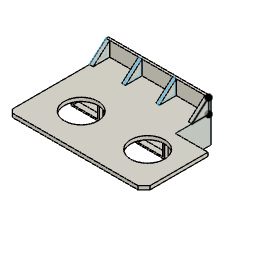
Magneto+Cooler+Gehäuse (Autodesk Fusion 360 design; units mm, degrees)
Autodesk Fusion 360 part; units mm, degrees
sketch "Skizze1" plane through (0, 0, 0) normal (0, 1, 0) x (1, 0, 0)
  line L0 (0, 0) -> (85, 0)
  line L1 (85, 0) -> (85, -25)
  line L2 (85, -25) -> (0, -25)
  line L3 (0, -25) -> (0, 0)
  line L4 (85, 0) -> (85, -10)
  line L5 (5, -10) -> (17, -10)
  line L6 (17, -10) -> (17, -19)
  line L7 (17, -19) -> (5, -19)
  line L8 (5, -19) -> (5, -10)
  line L9 (32, -19) -> (20, -19)
  line L10 (20, -19) -> (20, -10)
  line L11 (20, -10) -> (32, -10)
  line L12 (32, -10) -> (32, -19)
  line L13 (47, -19) -> (35, -19)
  line L14 (35, -19) -> (35, -10)
  line L15 (35, -10) -> (47, -10)
  line L16 (47, -10) -> (47, -19)
  line L17 (62, -19) -> (50, -19)
  line L18 (50, -19) -> (50, -10)
  line L19 (50, -10) -> (62, -10)
  line L20 (62, -10) -> (62, -19)
  line L21 (82, -19) -> (70, -19)
  line L22 (70, -19) -> (70, -10)
  line L23 (70, -10) -> (82, -10)
  line L24 (82, -10) -> (82, -19)
  line L25 (6.5, -11.5) -> (15.5, -11.5)
  line L26 (15.5, -11.5) -> (15.5, -17.5)
  line L27 (15.5, -17.5) -> (6.5, -17.5)
  line L28 (6.5, -17.5) -> (6.5, -11.5)
  line L29 (21.5, -11.5) -> (30.5, -11.5)
  line L30 (30.5, -11.5) -> (30.5, -17.5)
  line L31 (30.5, -17.5) -> (21.5, -17.5)
  line L32 (21.5, -17.5) -> (21.5, -11.5)
  line L33 (51.5, -11.5) -> (60.5, -11.5)
  line L34 (60.5, -11.5) -> (60.5, -17.5)
  line L35 (60.5, -17.5) -> (51.5, -17.5)
  line L36 (51.5, -17.5) -> (51.5, -11.5)
  line L37 (36.5, -11.5) -> (45.5, -11.5)
  line L38 (45.5, -11.5) -> (45.5, -17.5)
  line L39 (45.5, -17.5) -> (36.5, -17.5)
  line L40 (36.5, -17.5) -> (36.5, -11.5)
  line L41 (71.5, -11.5) -> (80.5, -11.5)
  line L42 (80.5, -11.5) -> (80.5, -17.5)
  line L43 (80.5, -17.5) -> (71.5, -17.5)
  line L44 (71.5, -17.5) -> (71.5, -11.5)
  dimension "d1" = 85
  dimension "d2" = 25
  dimension "d3" = 10
  dimension "d4" = 12
  dimension "d5" = 9
  dimension "d9" = 45
  dimension "d10" = 0
  dimension "d13" = 20
  dimension "d14" = 0
  dimension "d16" = 1.5
  dimension "d17" = 1.5
  dimension "d18" = 1.5
  dimension "d19" = 1.5
  dimension "d20" = 1.5
  constraint horizontal L0
  constraint vertical L1
  constraint horizontal L2
  constraint vertical L3
  constraint coincident L0.start L3.end
  constraint perpendicular L0 L4
  constraint horizontal L5
  constraint vertical L6
  constraint horizontal L7
  constraint vertical L8
  measures "d1" distance of L0.start L0.end
  measures "d2" distance of L0.start L2.end
  measures "d3" distance of L0.end L4.end
  measures "d4" distance of L5.start L5.end
  measures "d5" distance of L5.start L7.end
extrude "Extrusion1" add sketch "Skizze1" along normal blind 3 contours L0 L1 L2 L3 L4
extrude "Extrusion2" add sketch "Skizze1" along normal blind 5 contours L5 L6 L7 L8 | L9 L10 L11 L12 | L13 L14 L15 L16 | L17 L18 L19 L20 | L21 L22 L23 L24
sketch "Skizze2" plane through (0, 0, 0) normal (0, 1, 0) x (1, 0, 0)
  line L0 (0, -25) -> (85, -25)
  line L1 (85, -25) -> (85, 0)
  line L2 (85, 0) -> (0, 0)
  line L3 (0, 0) -> (0, -25)
  line L4 (83.5, -1.5) -> (1.5, -1.5)
  line L5 (1.5, -1.5) -> (1.5, -23.5)
  line L6 (1.5, -23.5) -> (83.5, -23.5)
  line L7 (83.5, -23.5) -> (83.5, -1.5)
  point P0 (0, -25)
  point P1 (85, 0)
  dimension "d25" = -1.5
  constraint horizontal L0
  constraint vertical L1
  constraint horizontal L2
  constraint vertical L3
  constraint coincident P1 L1.end
  constraint coincident P0 L0.start
extrude "Extrusion3" add sketch "Skizze2" against normal blind 25
sketch "Skizze3" plane through (0, -25, 0) normal (0, -1, 0) x (1, 0, 0)
  line L0 (83.5, 23.5) -> (83.5, 1.5)
  line L1 (83.5, 1.5) -> (1.5, 1.5)
  line L2 (1.5, 1.5) -> (1.5, 23.5)
  line L3 (1.5, 23.5) -> (83.5, 23.5)
  line L4 (0, 25) -> (0, 0)
  line L5 (0, 0) -> (85, 0)
  line L6 (85, 0) -> (85, 25)
  line L7 (85, 25) -> (0, 25)
  line L8 (0, 25) -> (85, 25)
  line L9 (85, 25) -> (85, 0)
  line L10 (85, 0) -> (0, 0)
  line L11 (0, 0) -> (0, 25)
  constraint horizontal L8
  constraint vertical L9
  constraint horizontal L10
  constraint vertical L11
  constraint coincident L5.end L6.start
  constraint coincident L4.start L7.end
extrude "Extrusion4" add sketch "Skizze3" along normal blind 1.5 contours L0 L1 L2 L3 | L4 L5 L6 L7 L8 L9 L10 L11
sketch "Skizze4" plane through (0, -26.5, 0) normal (0, -1, 0) x (1, 0, 0)
  line L0 (0, 0) -> (85, 0)
  line L1 (85, 0) -> (85, 25)
  line L2 (85, 25) -> (0, 25)
  line L3 (0, 25) -> (0, 0)
  line L4 (3, 20) -> (22.8, 20)
  line L5 (22.8, 20) -> (22.8, 4.6)
  line L6 (22.8, 4.6) -> (3, 4.6)
  line L7 (3, 4.6) -> (3, 20)
  line L8 (4.45, 5.8) -> (21.35, 5.8)
  line L9 (21.35, 5.8) -> (21.35, 18.8)
  line L10 (21.35, 18.8) -> (4.45, 18.8)
  line L11 (4.45, 18.8) -> (4.45, 5.8)
  line L12 (76.8, 4.6) -> (57, 4.6)
  line L13 (76.8, 20) -> (76.8, 4.6)
  line L14 (58.45, 18.8) -> (58.45, 5.8)
  line L15 (57, 20) -> (76.8, 20)
  line L16 (75.35, 5.8) -> (75.35, 18.8)
  line L17 (75.35, 18.8) -> (58.45, 18.8)
  line L18 (57, 4.6) -> (57, 20)
  line L19 (58.45, 5.8) -> (75.35, 5.8)
  line L20 (109, 20) -> (109, 23)
  line L21 (109, 23) -> (0, 23)
  line L22 (109, 20) -> (0, 20)
  line L23 (0, 23) -> (0, 20)
  dimension "d30" = 19.8
  dimension "d31" = 15.4
  dimension "d33" = 16.9
  dimension "d34" = 13
  dimension "d36" = 19.8
  dimension "d37" = 15.4
  dimension "d38" = 16.9
  dimension "d39" = 13
  dimension "d40" = 52
  dimension "d41" = 3
  constraint horizontal L4
  constraint vertical L5
  constraint horizontal L6
  constraint vertical L7
  constraint horizontal L8
  constraint vertical L9
  constraint horizontal L10
  constraint vertical L11
  constraint horizontal L15
  constraint vertical L13
  constraint horizontal L12
  constraint vertical L18
  constraint horizontal L19
  constraint vertical L16
  constraint horizontal L17
  constraint vertical L14
  constraint coincident L3 L21.end
  constraint perpendicular L3 L21
  constraint coincident L3 L22.end
  constraint perpendicular L3 L22
  measures "d30" distance of L4.start L4.end
  measures "d31" distance of L4.start L6.end
  measures "d33" distance of L8.start L8.end
  measures "d34" distance of L8.start L10.end
  measures "d36" distance of L15.start L13.start
  measures "d37" distance of L15.start L12.end
  measures "d38" distance of L16.start L14.end
  measures "d39" distance of L14.end L14.start
  measures "d40" distance of L15.start L20.start
  measures "d41" distance of L20.start L20.end
extrude "Extrusion5" cut sketch "Skizze4" against normal blind 3 contours L8 L9 L10 L11 | L14 L16 L17 L19
extrude "Extrusion6" add sketch "Skizze4" along normal blind 3 contours L4 L5 L6 L7 L22 | L12 L13 L15 L18 L22
extrude "Extrusion7" add sketch "Skizze4" along normal blind 53 contours L1 L3 L4 L15 L21 L22 L23 | L1 L20 L21 L22
sketch "Skizze5" plane through (0, 0, 23) normal (0, 0, 1) x (-1, 0, 0)
  line L0 (-109, 26.5) -> (-85, 26.5)
  line L1 (-85, 26.5) -> (0, 26.5)
  line L2 (0, 26.5) -> (0, 79.5)
  line L3 (0, 79.5) -> (-109, 79.5)
  line L4 (-109, 79.5) -> (-109, 26.5)
  line L5 (-85, 26.5) -> (-85, 79.5)
  line L6 (-85, 26.5, 2) -> (-85, 79.5, 0)
  line L7 (-85, 26.5, 2) -> (-85, 26.5, 0)
  line L8 (0, 26.5) -> (0, 79.5)
  line L9 (0, 26.5, 2) -> (0, 79.5, 0)
  line L10 (0, 26.5, 2) -> (0, 26.5, 0)
  point P0 (-85, 26.5)
  point P1 (0, 26.5)
  point P2 (0, 26.5)
  constraint coincident P0 L0.end
  constraint coincident L3 L5.end
  constraint perpendicular L3 L5
  constraint coincident P2 P1
  constraint coincident L2.end L3.start
extrude "Extrusion8" add sketch "Skizze5" against normal blind 3 contours L2 L8 L9 L10 in plane through (0, 0, 23) normal (-1, 0, 0)
extrude "Extrusion9" add sketch "Skizze5" along normal blind 3 contours L5 L6 L7 in plane through (85, 0, 23) normal (-1, 0, 0)
extrude "Extrusion10" cut 5 faces at (78, 3.6667, 19) (58, 3.6667, 19) (43, 3.6667, 19) (28, 3.6667, 19) (13, 3.6667, 19) along direction (0, 0, -1) blind 0.5
extrude "Extrusion11" cut 5 faces at (74, 3.6667, 10) (54, 3.6667, 10) (39, 3.6667, 10) (24, 3.6667, 10) (9, 3.6667, 10) along direction (0, 0, 1) blind 0.5
extrude "Extrusion12" cut 1 faces at (17, 3.6667, 13.1667) along direction (-1, 0, 0) blind 0.5
extrude "Extrusion13" cut 1 faces at (32, 3.6667, 13.1667) along direction (-1, 0, 0) blind 0.5
extrude "Extrusion14" cut 1 faces at (47, 3.6667, 13.1667) along direction (-1, 0, 0) blind 0.5
extrude "Extrusion15" cut 1 faces at (62, 3.6667, 13.1667) along direction (-1, 0, 0) blind 0.5
extrude "Extrusion16" cut 1 faces at (82, 3.6667, 13.1667) along direction (-1, 0, 0) blind 0.5
extrude "Extrusion17" cut 1 faces at (70, 3.6667, 15.8333) along direction (1, 0, 0) blind 0.5
extrude "Extrusion18" cut 1 faces at (50, 3.6667, 15.8333) along direction (1, 0, 0) blind 0.5
extrude "Extrusion19" cut 1 faces at (35, 3.6667, 15.8333) along direction (1, 0, 0) blind 0.5
extrude "Extrusion20" cut 1 faces at (20, 3.6667, 15.8333) along direction (1, 0, 0) blind 0.5
extrude "Extrusion21" cut 1 faces at (5, 3.6667, 15.8333) along direction (1, 0, 0) blind 0.5
extrude "Extrusion22" add 5 faces at (77.5, 5, 18.1667) (57.5, 5, 18.1667) (42.5, 5, 18.1667) (27.5, 5, 18.1667) (9.5, 5, 18.1667) along direction (0, 1, 0) blind 1
extrude "Extrusion23" cut 1 faces at (69.7167, -28, 18.8) along direction (0, 0, 1) blind 1
extrude "Extrusion24" cut 1 faces at (15.7167, -28, 18.8) along direction (0, 0, 1) blind 1
extrude "Extrusion25" add 1 faces at (22.8, -27.5, 14.8667) along direction (1, 0, 0) blind 1.2
extrude "Extrusion26" add 1 faces at (76.8, -27.5, 14.8667) along direction (1, 0, 0) blind 1.2
extrude "Extrusion27" cut 1 faces at (75.35, -26.5, 10.4667) along direction (1, 0, 0) blind 1.2
extrude "Extrusion28" cut 1 faces at (21.35, -26.5, 10.4667) along direction (1, 0, 0) blind 1.2
extrude "Extrusion29" add 1 faces at (17, -28.5, 4.6) along direction (0, 0, -1) blind 1.2
extrude "Extrusion30" add 1 faces at (71, -28.5, 4.6) along direction (0, 0, -1) blind 1.2
extrude "Extrusion31" cut 1 faces at (16.5167, -28, 5.8) along direction (0, 0, -1) blind 1.2
extrude "Extrusion32" cut 1 faces at (70.5167, -28, 5.8) along direction (0, 0, -1) blind 1.2
extrude "Extrusion33" add 1 faces at (57, -27.5, 8.9333) along direction (-1, 0, 0) blind 1.2
extrude "Extrusion34" add 1 faces at (3, -27.5, 8.9333) along direction (-1, 0, 0) blind 1.2
extrude "Extrusion35" cut 1 faces at (4.45, -26.5, 9.6667) along direction (-1, 0, 0) blind 1.2
extrude "Extrusion36" cut 1 faces at (58.45, -28, 9.6667) along direction (-1, 0, 0) blind 1.2
extrude "Extrusion37" add 1 faces at (78, -27.5, 14.4667) along direction (1, 0, 0) blind 1
extrude "Extrusion38" cut 1 faces at (76.55, -28, 14.7333) along direction (1, 0, 0) blind 1
extrude "Extrusion39" add 1 faces at (24, -27.5, 14.4667) along direction (1, 0, 0) blind 1
extrude "Extrusion40" cut 1 faces at (22.55, -28, 9.6667) along direction (1, 0, 0) blind 1
extrude "Extrusion41" add 1 faces at (71.2667, -28.5, 3.4) along direction (0, 0, -1) blind 0.5
extrude "Extrusion42" add 1 faces at (17.2667, -28.5, 3.4) along direction (0, 0, -1) blind 0.5
extrude "Extrusion43" cut 1 faces at (64.0167, -28, 4.6) along direction (0, 0, -1) blind 0.5
extrude "Extrusion44" cut 1 faces at (16.7833, -28, 4.6) along direction (0, 0, -1) blind 0.5
extrude "Extrusion45" cut 1 faces at (3, -44.1667, 23.6667) along direction (-1, 0, 0) blind 15
extrude "Extrusion46" cut 1 faces at (82, -44.1667, 23.6667) along direction (1, 0, 0) blind 25
extrude "Extrusion47" cut 1 faces at (56.6667, -16.6667, 25) along direction (0, 0, -1) blind 2
sketch "Skizze6" plane through (0, 0, 23) normal (0, 0, 1) x (-1, 0, 0)
  line L0 (-83.5, 25) -> (-1.5, 25)
  line L1 (-1.5, 25) -> (-1.5, 0)
  line L2 (-1.5, 0) -> (-83.5, 0)
  line L3 (-83.5, 0) -> (-83.5, 25)
  line L4 (0, -3) -> (0, 79.5)
  line L5 (0, 79.5) -> (-109, 79.5)
  line L6 (-109, 79.5) -> (-109, 26.5)
  line L7 (-109, 26.5) -> (-85, 26.5)
  line L8 (-85, 26.5) -> (-85, -3)
  line L9 (-85, -3) -> (0, -3)
  line L10 (-1.5, 0) -> (-83.5, 0)
  line L11 (-83.5, 0) -> (-83.5, 25)
  line L12 (-83.5, 25) -> (-1.5, 25)
  line L13 (-1.5, 25) -> (-1.5, 0)
  constraint horizontal L10
  constraint vertical L11
  constraint horizontal L12
  constraint vertical L13
  constraint coincident L0.start L3.end
  constraint coincident L1.end L2.start
extrude "Extrusion48" add sketch "Skizze6" against normal blind 2 contours L0 L1 L2 L3 L10 L11 L12 L13
extrude "Extrusion49" add 1 faces at (109, -44.1667, 21) along direction (1, 0, 0) blind 3
chamfer "Fase1" distance 5 angle 45 1 edges at (112, -79.5, 21.5)
chamfer "Fase2" distance 3 angle 45 1 edges at (0, -79.5, 21.5)
sketch "Skizze7" plane through (0, 0, 23) normal (0, 0, 1) x (-1, 0, 0)
  line L0 (0, 76.5) -> (-3, 79.5)
  line L1 (-3, 79.5) -> (-107, 79.5)
  line L2 (-107, 79.5) -> (-112, 74.5)
  line L3 (-112, 74.5) -> (-112, 26.5)
  line L4 (-112, 26.5) -> (-85, 26.5)
  line L5 (-85, 26.5) -> (-85, -3)
  line L6 (-85, -3) -> (0, -3)
  line L7 (0, -3) -> (0, 76.5)
  circle A0 centre (-30, 49.5) radius 14
  circle A1 centre (-85, 49.5) radius 14
  dimension "d136" = 28
  dimension "d137" = 28
  measures "d136" diameter of A0
  measures "d137" diameter of A1
extrude "Extrusion50" cut sketch "Skizze7" against normal blind 5 contours A0 | A1
sketch "Skizze8" plane through (0, 0, 23) normal (0, 0, 1) x (-1, 0, 0)
  circle A0 centre (-30, 49.5) radius 14
  circle A1 centre (-85, 49.5) radius 14
  line L0 (0, 76.5) -> (-3, 79.5)
  line L1 (-3, 79.5) -> (-107, 79.5)
  line L2 (-107, 79.5) -> (-112, 74.5)
  line L3 (-112, 74.5) -> (-112, 26.5)
  line L4 (-112, 26.5) -> (-85, 26.5)
  line L5 (-85, 26.5) -> (-85, -3)
  line L6 (-85, -3) -> (0, -3)
  line L7 (0, -3) -> (0, 76.5)
  line L8 (0, -3) -> (-85, -3)
  line L9 (-85, -3) -> (-85, -1)
  line L10 (-85, -1) -> (0, -1)
  line L11 (0, -1) -> (0, -3)
  dimension "d140" = 2
  constraint horizontal L8
  constraint vertical L9
  constraint horizontal L10
  constraint vertical L11
  constraint coincident L6.end L7.start
  measures "d140" distance of L6.end L10.end
extrude "Extrusion51" add sketch "Skizze8" along normal blind 12 contours L5 L6 L7 L8 L9 L10 L11
sketch "Skizze9" plane through (85, 0, 0) normal (1, 0, 0) x (0, 1, 0)
  line L0 (1, 23) -> (-26.5, 23)
  line L1 (-26.5, 23) -> (-26.5, 20)
  line L2 (-26.5, 20) -> (-26.5, 0)
  line L3 (-26.5, 0) -> (3, 0)
  line L4 (3, 0) -> (3, 35)
  line L5 (3, 35) -> (1, 35)
  line L6 (1, 35) -> (1, 23)
  line L7 (1, 35) -> (1, 23)
  line L8 (1, 35) -> (-12.75, 23)
  line L9 (1, 23) -> (-12.75, 23)
  line L10 (1, 35, -28.3) -> (-12.75, 23, -28.3)
  line L11 (1, 35, -28.3) -> (1, 23, -28.3)
  line L12 (1, 23, -28.3) -> (-12.75, 23, -28.3)
  line L13 (1, 35, -56.6) -> (-12.75, 23, -56.6)
  line L14 (1, 35, -56.6) -> (1, 23, -56.6)
  line L15 (1, 23, -56.6) -> (-12.75, 23, -56.6)
  line L16 (1, 35, -84.9) -> (-12.75, 23, -84.9)
  line L17 (1, 35, -84.9) -> (1, 23, -84.9)
  line L18 (1, 23, -84.9) -> (-12.75, 23, -84.9)
  constraint coincident L5.end L6.start
  constraint coincident L0.start L6.end
  constraint midpoint L0 L8.end
extrude "Extrusion52" add sketch "Skizze9" against normal blind 3 contours L0 L6 L7 L8 L9
extrude "Extrusion53" add sketch "Skizze9" along normal blind 3 contours L16 L17 L18 in plane through (0.1, 0, 0) normal (1, 0, 0)
extrude "Extrusion54" add sketch "Skizze9" along normal mid plane 3 contours L13 L14 L15 in plane through (28.4, 0, 0) normal (1, 0, 0)
extrude "Extrusion55" add sketch "Skizze9" along normal mid plane 3 contours L10 L11 L12 in plane through (56.7, 0, 0) normal (1, 0, 0)
equation "d13 = 8 mm + 12 mm"
